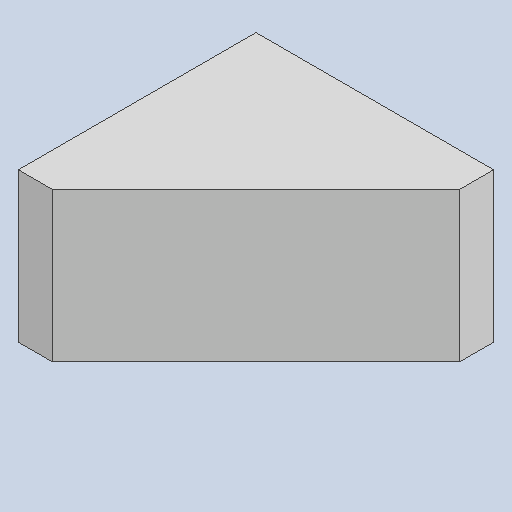
# Autodesk Inventor part: Union_Inferior
Saved by Autodesk Inventor 2024 (Build 280153000, 153)
## iProperties
Created: 2024-07-16
Part Number: Union_Inferior
Material: Genérico
Document SubType Name: Modeling
Designer: sergi
Density: 1 g/cm^3
Appearance: Valor por defecto
Author: sergi
Autodesk Inventor part; units mm, degrees
ref_plane "YZ Plane" through (0, 0, 0) normal (1, 0, 0) x (0, 1, 0)
ref_plane "XZ Plane" through (0, 0, 0) normal (0, 1, 0) x (-1, 0, 0)
ref_plane "XY Plane" through (0, 0, 0) normal (0, 0, 1) x (1, 0, 0)
sketch "Boceto1" plane through (0, 0, 0) normal (0, 0, 1) x (1, 0, 0)
  circle A0 centre (88, 48.5) radius 1.5 projected
  circle A1 centre (88, -51.5) radius 1.5 projected
  circle A2 centre (-50, 86.5) radius 1.5 projected
  circle A3 centre (50, 86.5) radius 1.5 projected
  circle A4 centre (-88, -51.5) radius 1.5 projected
  circle A5 centre (-88, 48.5) radius 1.5 projected
  circle A6 centre (50, -89.5) radius 1.5 projected
  circle A7 centre (-50, -89.5) radius 1.5 projected
  line L0 (-103, -104.5) -> (-103, 101.5) projected
  line L1 (103, -104.5) -> (-103, -104.5) projected
  line L2 (103, 101.5) -> (103, -104.5) projected
  line L3 (-100, -104.5) -> (-100, 89.3) projected
  line L4 (-88, -51.5) -> (-100, -51.5)
  line L5 (-88, -51.5) -> (-82.5, -51.5)
  line L6 (-82.5, -51.5) -> (-82.5, -57)
  line L7 (-82.5, -57) -> (-100, -57)
  line L8 (-100, -57) -> (-100, -46)
  line L9 (-100, -46) -> (-82.5, -46)
  line L10 (-82.5, -46) -> (-82.5, -57)
  circle A8 centre (-88, -51.5) radius 2.1
  line L11 (-103, 101.5) -> (103, 101.5) projected
  point P0 (0, 0)
  dimension "d0" = 5.5
  dimension "d1" = 5.5
  dimension "d2" = 11
  dimension "d14" = 4.2
  constraints: 14 end point, 2 horizontal, 2 parallel, 2 perpendicular, 2 point on line, 1 centre point, 1 coincident, 1 vertical
  measures "d0" distance of L4.start L5.end
  measures "d1" distance of L5.end L6.end
  measures "d2" distance of L7.end L8.end
  measures "d14" diameter of A8
extrude "Extrusión1" add sketch "Boceto1" along normal blind 17.5 contours L5 L4 A4 | L5 A8 L4 A4 | A4 L4 L5 | A4 L4 A8 L5 | A8 L4 L3 L9 L10 L5 | L5 L6 L7 L3 L4 A8
sketch "Boceto2" plane through (-100, -57, 0) normal (-1, 0, 0) x (0, 0, 1)
  line L0 (0, 0) -> (17.5, 0) projected
  line L1 (0, 11) -> (0, 0) projected
  point P0 (0, 57)
  point P1 (12, 5.5)
  dimension "d5" = 5.5
  dimension "d6" = 12
  measures "d5" distance from line of L0 point (12, 5.5)
  measures "d6" distance from line of L1 point (12, 5.5)
hole "Agujero1" at (-100, -51.5, 12) direction (1, 0, 0) diameter 4.2 depth 4
sketch "Boceto3" plane through (0, 0, 0) normal (0, 0, -1) x (-1, 0, 0)
  line L0 (100, -46) -> (100, -57) projected
  line L1 (82.5, -46) -> (100, -46) projected
  point P0 (0, 0)
  point P1 (88, -51.5)
  dimension "d15" = 12
  dimension "d16" = 5.5
  measures "d15" distance from line of L0 point (88, -51.5)
  measures "d16" distance from line of L1 point (88, -51.5)
hole "Agujero2" at (-88, -51.5, 0) direction (0, 0, 1) diameter 4.2 depth 4
chamfer "Chaflán1" distance 15 angle 45 1 edges at (-82.5, -51.5, 17.5)
